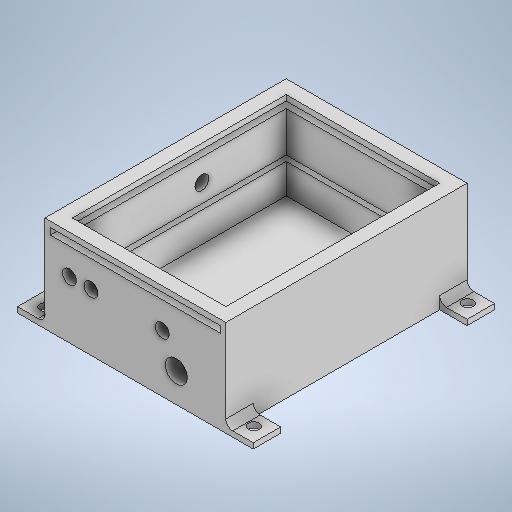
# Autodesk Inventor part: Housing
Saved by Autodesk Inventor 2025 (Build 290162000, 162)
## iProperties
Created: 2024-10-01
Part Number: Housing
Material: Generic
Document SubType Name: Modeling
Designer: willi
Density: 1 g/cm^3
Appearance: Default
Author: willi
Autodesk Inventor part; units mm, degrees
ref_plane "YZ Plane" through (0, 0, 0) normal (1, 0, 0) x (0, 1, 0)
ref_plane "XZ Plane" through (0, 0, 0) normal (0, 1, 0) x (-1, 0, 0)
ref_plane "XY Plane" through (0, 0, 0) normal (0, 0, 1) x (1, 0, 0)
sketch "Sketch1" plane through (0, 0, 0) normal (0, 1, 0) x (-1, 0, 0)
  line L0 (31.1869, 36.5935) -> (-39.9331, 36.5935)
  line L1 (-39.9331, 36.5935) -> (-39.9331, -62.4665)
  line L2 (-39.9331, -62.4665) -> (31.1869, -62.4665)
  line L3 (31.1869, -62.4665) -> (31.1869, 36.5935)
  line L4 (37.5369, 42.9435) -> (-46.2831, 42.9435)
  line L5 (-46.2831, 42.9435) -> (-46.2831, -68.8165)
  line L6 (-46.2831, -68.8165) -> (37.5369, -68.8165)
  line L7 (37.5369, -68.8165) -> (37.5369, 42.9435)
  line L8 (28.6469, 34.0535) -> (-37.3931, 34.0535)
  line L9 (-37.3931, 34.0535) -> (-37.3931, -59.9265)
  line L10 (-37.3931, -59.9265) -> (28.6469, -59.9265)
  line L11 (28.6469, -59.9265) -> (28.6469, 34.0535)
  point P0 (0, 0)
  point P1 (-4.3731, -62.4665)
  point P2 (-4.3731, 36.5935)
  dimension "d0" = 71.12
  dimension "d1" = 99.06
  dimension "d2" = 6.35
  dimension "d3" = 6.35
  dimension "d4" = 6.35
  dimension "d5" = 6.35
  dimension "d22" = 2.54
  dimension "d23" = 2.54
  dimension "d24" = 2.54
  dimension "d25" = 2.54
  constraints: 24 end point, 6 parallel, 3 horizontal, 3 perpendicular, 2 midpoint
  measures "d0" distance of L1.end L2.end
  measures "d1" distance of L2.end L0.start
  measures "d2" distance between parallel lines of L7 L3
  measures "d3" distance between parallel lines of L4 L0
  measures "d4" distance between parallel lines of L5 L1
  measures "d5" distance between parallel lines of L2 L6
  measures "d22" distance between parallel lines of L3 L11
  measures "d23" distance between parallel lines of L10 L2
  measures "d24" distance between parallel lines of L9 L1
  measures "d25" distance between parallel lines of L8 L0
extrude "Extrusion1" add sketch "Sketch1" against normal blind 44.45 contours L3 L2 L1 L0 | L7 L6 L5 L4 | L11 L10 L9 L8
extrude "Extrusion3" cut sketch "Sketch1" against normal blind 38.1 contours L11 L10 L9 L8
extrude "Extrusion4" cut sketch "Sketch1" against normal blind 24.257 contours L3 L2 L1 L0 | L11 L10 L9 L8
sketch "Sketch5" plane through (-37.5369, 0, 42.9435) normal (0, 0, 1) x (1, 0, 0)
  line L0 (2.54, -2.54) -> (81.28, -2.54)
  line L1 (81.28, -2.54) -> (81.28, -5.588)
  line L2 (81.28, -5.588) -> (2.54, -5.588)
  line L3 (2.54, -5.588) -> (2.54, -2.54)
  line L4 (0, 0) -> (83.82, 0) projected
  line L5 (83.82, 0) -> (83.82, -44.45) projected
  line L6 (0, 0) -> (0, -44.45) projected
  point P0 (37.5369, 0)
  point P1 (81.28, -4.064)
  point P2 (2.54, -4.064)
  dimension "d32" = 2.54
  dimension "d33" = 2.54
  dimension "d34" = 2.54
  dimension "d35" = 3.048
  constraints: 8 end point, 2 midpoint, 2 parallel, 1 horizontal, 1 perpendicular
  measures "d32" distance between parallel lines of L0 L4
  measures "d33" distance from line of L5 point (81.28, -4.064)
  measures "d34" distance from line of L6 point (2.54, -4.064)
  measures "d35" distance between parallel lines of L0 L2
extrude "Extrusion6" cut sketch "Sketch5" against normal blind 108.585
sketch "Sketch6" plane through (39.9331, -24.257, 36.5935) normal (0, 0, -1) x (-1, 0, 0)
  line L0 (71.12, 18.669) -> (71.12, 0) projected
  line L1 (0, 0) -> (71.12, 0) projected
  point P0 (39.9331, 24.257)
  point P1 (66.12, 6.35)
  point P2 (56.12, 6.35)
  point P3 (23.12, 6.35)
  point P4 (71.12, 9.3345)
  dimension "d38" = 5
  dimension "d39" = 15
  dimension "d40" = 48
  dimension "d41" = 6.35
  dimension "d42" = 6.35
  dimension "d43" = 6.35
  constraints: 1 midpoint
  measures "d38" horizontal distance of point (71.12, 9.334) point (66.12, 6.35)
  measures "d39" distance from line of L0 point (56.12, 6.35)
  measures "d40" distance from line of L0 point (23.12, 6.35)
  measures "d41" distance from line of L1 point (66.12, 6.35)
  measures "d42" distance from line of L1 point (56.12, 6.35)
  measures "d43" distance from line of L1 point (23.12, 6.35)
sketch "Sketch7" plane through (37.3931, -38.1, 34.0535) normal (0, 0, -1) x (-1, 0, 0)
  point P0 (37.3931, 38.1)
  point P1 (14.0713, 7.0927)
hole "Hole1" at (-26.1869, -17.907, 36.5935) at (-16.1869, -17.907, 36.5935) at (16.8131, -17.907, 36.5935) direction (0, 0, 1) diameter 6.35 end through all
hole "Hole2" at (23.3218, -31.0073, 34.0535) direction (0, 0, 1) diameter 10.16 end through all
sketch "Sketch8" plane through (-31.1869, -24.257, 36.5935) normal (1, 0, 0) x (0, 0, -1)
  line L0 (0, 18.669) -> (0, 0) projected
  point P0 (36.5935, 24.257)
  point P1 (60, 8.5086)
  point P2 (0, 9.3345)
  dimension "d58" = 60
  constraints: 1 midpoint
  measures "d58" horizontal distance of point (0, 9.334) point (60, 8.509)
hole "Hole3" at (-31.1869, -15.7484, -23.4065) direction (-1, 0, 0) diameter 6.35 end through all
sketch "Sketch9" plane through (46.2831, 0, 42.9435) normal (1, 0, 0) x (0, 0, -1)
  line L0 (0, 0) -> (0, -44.45) projected
  line L1 (111.76, -44.45) -> (0, -44.45) projected
  line L2 (0, -41.91) -> (12.7, -41.91)
  line L3 (12.7, -41.91) -> (12.7, -44.45)
  line L4 (12.7, -44.45) -> (0, -44.45)
  line L5 (0, -44.45) -> (0, -41.91)
  line L6 (111.76, -41.91) -> (99.06, -41.91)
  line L7 (99.06, -41.91) -> (99.06, -44.45)
  line L8 (99.06, -44.45) -> (111.76, -44.45)
  line L9 (111.76, -44.45) -> (111.76, -41.91)
  line L10 (111.76, 0) -> (111.76, -44.45) projected
  point P0 (42.9435, 0)
  point P1 (111.76, -43.18)
  dimension "d66" = 12.7
  dimension "d67" = 12.7
  dimension "d68" = 0
  dimension "d69" = 2.54
  dimension "d70" = 2.54
  constraints: 16 end point, 4 parallel, 3 point on line, 2 horizontal, 2 perpendicular, 1 midpoint
  measures "d66" distance of L2.start L2.end
  measures "d67" distance of L6.start L6.end
  measures "d68" distance from line of L10 point (111.76, -43.18)
  measures "d69" distance of L6.end L7.end
  measures "d70" distance of L2.end L3.end
extrude "Extrusion7" add sketch "Sketch9" along normal blind 12.7
sketch "Sketch10" plane through (46.2831, -41.91, 42.9435) normal (0, 1, 0) x (1, 0, 0)
  point P0 (-46.2831, 42.9435)
  point P1 (6.2127, 6.7401)
  point P2 (6.4208, 105.6569)
hole "Hole4" at (52.4958, -41.91, 36.2034) at (52.7039, -41.91, -62.7134) direction (0, -1, 0) diameter 5.08 end through all clearance for "Flat Head Machine Screw (82)" size "#8" standard "Ansi Unified Screw Threads"
fillet "Fillet1" radius 3.175 2 edges at (46.2831, -41.91, 36.5935) (46.2831, -41.91, -62.4665)
sketch "Sketch11" plane through (-37.5369, 0, -68.8165) normal (-1, 0, 0) x (0, 0, 1)
  line L0 (0, -41.91) -> (12.7, -41.91) projected
  line L1 (12.7, -41.91) -> (12.7, -44.45) projected
  line L2 (0, -41.91) -> (12.7, -41.91)
  line L3 (12.7, -41.91) -> (12.7, -44.45)
  line L4 (12.7, -44.45) -> (0, -44.45)
  line L5 (0, -44.45) -> (0, -41.91)
  line L6 (111.76, -41.91) -> (111.76, -44.45) projected
  line L7 (99.06, -38.735) -> (99.06, -44.45) projected
  line L8 (111.76, -44.45) -> (99.06, -44.45)
  line L9 (99.06, -44.45) -> (99.06, -41.91)
  line L10 (99.06, -41.91) -> (111.76, -41.91)
  line L11 (111.76, -41.91) -> (111.76, -44.45)
  point P0 (68.8165, 0)
  constraints: 16 end point, 4 parallel, 2 horizontal, 2 perpendicular, 2 point on line
extrude "Extrusion8" add sketch "Sketch11" along normal blind 12.7
sketch "Sketch12" plane through (-37.5369, -41.91, -56.1165) normal (0, 1, 0) x (1, 0, 0)
  point P0 (37.5369, -56.1165)
  point P1 (-6.2476, 6.7674)
  point P2 (-5.9874, -92.7423)
hole "Hole5" at (-43.7845, -41.91, -62.8839) at (-43.5243, -41.91, 36.6258) direction (0, -1, 0) diameter 5.08 end through all clearance for "Flat Head Machine Screw (82)" size "#8" standard "Ansi Unified Screw Threads"
fillet "Fillet2" radius 3.175 2 edges at (-37.5369, -41.91, -62.4665) (-37.5369, -41.91, 36.5935)
body "Solid1"
